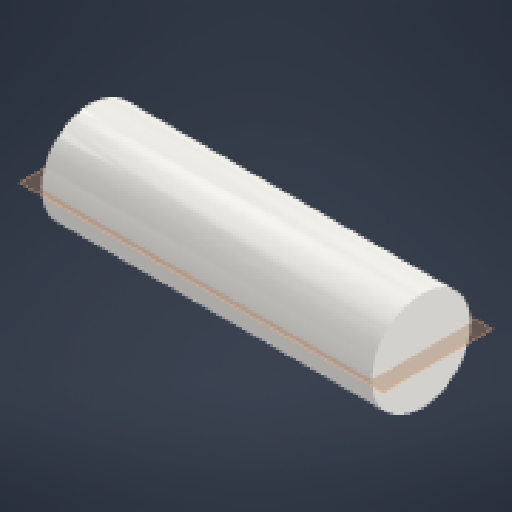
# Autodesk Inventor part: ArbreRoue
Saved by Autodesk Inventor 2026.2 (Build 302298010, 298A)
## iProperties
Created: 2026-03-31
Part Number: ArbreRoue
Material: Steel
Document SubType Name: Modeling
Designer: romai
Density: 1 g/cm^3
Appearance: Steel
CustomPartVersion: 1
Author: romai
Length: 150,000 mm
Autodesk Inventor part; units mm, degrees
ref_plane "Plan de départ" through (0, 0, 0) normal (1, 0, 0) x (0, 1, 0)
ref_plane "XY Plane" through (0, 0, 0) normal (0, 0, 1) x (1, 0, 0)
sketch "Esquisse principale" plane through (0, 0, 0) normal (0, 0, 1) x (1, 0, 0)
  line L0 (0, 0) -> (150, 0)
  line L1 (0, 0) -> (0, 12)
  line L2 (150, 12) -> (150, 0)
  line L3 (0, 12) -> (150, 12)
  dimension "d3" = 24
  constraints: 8 end point, 2 horizontal, 2 vertical
  measures "d3" diameter of L3 L0
revolve "Révolution1" add sketch "Esquisse principale" angle 360 about axis through (0, 0, 0) along (1, 0, 0)
equation "\"Length\" = 150"
